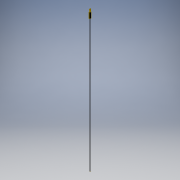
# Autodesk Inventor part: plug
Saved by Autodesk Inventor 2016 (Build 200138000, 138)
## iProperties
Created: 2017-02-28
Part Number: plug
Material: Generic
Document SubType Name: Modeling
Designer: 170007
Density: 1 g/cm^3
Appearance: Gold - Metal
Author: 170007
Autodesk Inventor part; units mm, degrees
ref_plane "YZ Plane" through (0, 0, 0) normal (1, 0, 0) x (0, 1, 0)
ref_plane "XZ Plane" through (0, 0, 0) normal (0, 1, 0) x (-1, 0, 0)
ref_plane "XY Plane" through (0, 0, 0) normal (0, 0, 1) x (1, 0, 0)
sketch "Sketch1" plane through (0, 0, 0) normal (0, 1, 0) x (-1, 0, 0)
  circle A0 centre (2.4819, 9.1831) radius 0.635
  point P0 (0, 0)
  dimension "d0" = 1.27
  constraints: 1 centre point
  measures "d0" diameter of A0
extrude "Extrusion1" add sketch "Sketch1" along normal blind 304.8
sketch "Sketch2" plane through (-2.4819, 304.8, 9.1831) normal (0, 1, 0) x (1, 0, 0)
  line L0 (-1.0816, -1.7196) -> (0.8833, -1.7196)
  line L1 (0.8833, -1.7196) -> (0.8833, 1.4308)
  line L2 (0.8833, 1.4308) -> (-1.0816, 1.4308)
  line L3 (-1.0816, 1.4308) -> (-1.0816, -1.7196)
  point P0 (2.4819, 9.1831)
  constraints: 8 end point, 2 parallel, 1 horizontal, 1 perpendicular
extrude "Extrusion2" add sketch "Sketch2" along normal blind 12.7
sketch "Sketch3" plane through (-2.4819, 317.5, 9.1831) normal (0, 1, 0) x (1, 0, 0)
  line L0 (-0.7645, -1.2984) -> (0.6263, -1.2984)
  line L1 (0.6263, -1.2984) -> (0.6263, -1.1087)
  line L2 (0.6263, -1.1087) -> (-0.7645, -1.1087)
  line L3 (-0.7645, -1.1087) -> (-0.7645, -1.2984)
  line L4 (-0.7645, 0.6885) -> (0.5541, 0.6885)
  line L5 (0.5541, 0.6885) -> (0.5541, 0.8962)
  line L6 (0.5541, 0.8962) -> (-0.7645, 0.8962)
  line L7 (-0.7645, 0.8962) -> (-0.7645, 0.6885)
  point P0 (2.4819, 9.1831)
  constraints: 16 end point, 4 parallel, 2 horizontal, 2 perpendicular, 1 point on line
extrude "Extrusion3" add sketch "Sketch3" along normal blind 6.35
body "Solid1"
